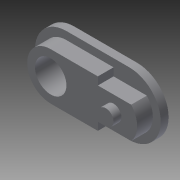
# Autodesk Inventor part: HW 6 Part 6
Saved by Autodesk Inventor 2015 (Build 190159000, 159)
## iProperties
Created: 2016-02-13
Part Number: HW 6 Part 6
Material: Generic
Document SubType Name: Modeling
Designer: Melissa
Density: 1 g/cm^3
Appearance: Default
Author: Melissa
Autodesk Inventor part; units mm, degrees
ref_plane "YZ Plane" through (0, 0, 0) normal (1, 0, 0) x (0, 1, 0)
ref_plane "XZ Plane" through (0, 0, 0) normal (0, 1, 0) x (-1, 0, 0)
ref_plane "XY Plane" through (0, 0, 0) normal (0, 0, 1) x (1, 0, 0)
sketch "Sketch1" plane through (0, 0, 0) normal (0, 0, 1) x (1, 0, 0)
  arc A0 (0, 25.4) -> (0, -25.4) centre (0, 0) ccw
  arc A1 (50.8, -25.4) -> (50.8, 25.4) centre (50.8, 0) ccw
  line L0 (0, 25.4) -> (50.8, 25.4)
  line L1 (0, -25.4) -> (50.8, -25.4)
  dimension "d2" = 50.8
  dimension "d3" = 50.8
  dimension "d4" = 50.8
  constraints: 4 end point, 4 point on circle, 3 tangent, 2 centre point, 2 horizontal, 1 coincident
  measures "d2" diameter of A0
  measures "d3" diameter of A1
  measures "d4" distance of A1.centre point (0, 0)
extrude "Extrusion1" add sketch "Sketch1" along normal blind 6.35
sketch "Sketch2" plane through (0, 0, 6.35) normal (0, 0, 1) x (1, 0, 0)
  arc A0 (0, 25.4) -> (0, -25.4) centre (0, 0) ccw projected
  line L0 (0, -25.4) -> (50.8, -25.4) projected
  arc A1 (50.8, -25.4) -> (50.8, 25.4) centre (50.8, 0) ccw projected
  line L1 (50.8, 25.4) -> (0, 25.4) projected
  arc A2 (0, 19.05) -> (0, -19.05) centre (0, 0) ccw
  arc A3 (64.999, -12.7) -> (64.999, 12.7) centre (50.8, 0) ccw
  line L2 (0, -19.05) -> (38.1, -19.05)
  line L3 (0, 19.05) -> (38.1, 19.05)
  line L4 (64.999, -12.7) -> (38.1, -12.7)
  line L5 (64.999, 12.7) -> (38.1, 12.7)
  circle A4 centre (0, 0) radius 12.7
  line L6 (38.1, 19.05) -> (38.1, 12.7)
  line L7 (38.1, -12.7) -> (38.1, -19.05)
  dimension "d8" = 38.1
  dimension "d9" = 38.1
  dimension "d10" = 38.1
  dimension "d11" = 38.1
  dimension "d16" = 25.4
  dimension "d17" = 25.4
  constraints: 12 end point, 4 perpendicular, 4 point on circle, 3 centre point, 3 coincident, 2 horizontal, 1 parallel, 1 tangent
  measures "d8" diameter of A2
  measures "d9" diameter of A3
  measures "d10" distance of L2.start L2.end
  measures "d11" distance of L3.start L3.end
  measures "d16" distance between parallel lines of L4 L5
  measures "d17" diameter of A4
extrude "Extrusion2" add sketch "Sketch2" along normal blind 12.7 contours L3 L6 L5 A3 L4 L7 L2 A2
sketch "Sketch3" plane through (0, 0, 6.35) normal (0, 0, 1) x (1, 0, 0)
  circle A0 centre (0, 0) radius 12.7
  dimension "d20" = 25.4
  constraints: 1 centre point, 1 coincident
  measures "d20" diameter of A0
extrude "Extrusion3" cut sketch "Sketch3" against normal through all
sketch "Sketch4" plane through (0, 0, 19.05) normal (0, 0, 1) x (1, 0, 0)
  circle A0 centre (0, 0) radius 12.7 projected
  arc A1 (0, 19.05) -> (0, -19.05) centre (0, 0) ccw projected
  line L0 (0, -19.05) -> (38.1, -19.05) projected
  line L1 (38.1, -19.05) -> (38.1, -12.7) projected
  line L2 (38.1, -12.7) -> (64.999, -12.7) projected
  arc A2 (64.999, -12.7) -> (64.999, 12.7) centre (50.8, 0) ccw projected
  line L3 (64.999, 12.7) -> (38.1, 12.7) projected
  line L4 (38.1, 12.7) -> (38.1, 19.05) projected
  line L5 (38.1, 19.05) -> (0, 19.05) projected
  circle A3 centre (50.8, 0) radius 6.35
  dimension "d23" = 12.7
  constraints: 1 centre point, 1 coincident
  measures "d23" diameter of A3
extrude "Extrusion4" add sketch "Sketch4" along normal blind 6.35 contours A3
body "Solid1"
